Autodesk Fusion 360 part; units mm, degrees
(part 5 of 6)
sketch "taco_truck" plane through (0, 0, 0) normal (0, 1, 0) x (1, 0, 0)
  line L0 (88.25, -7) -> (102.25, -7)
  line L1 (7, -7) -> (7, 7)
  line L2 (83.2, -7) -> (83.2, 7)
  line L3 (-7, 7) -> (-7, -7)
  line L4 (178.45, 7) -> (164.45, 7)
  line L5 (12.05, -7) -> (26.05, -7)
  line L6 (102.25, -7) -> (102.25, 7)
  line L7 (102.25, 7) -> (88.25, 7)
  line L8 (88.25, 7) -> (88.25, -7)
  line L9 (126.35, 7) -> (126.35, -7)
  line L10 (197.5, -7) -> (197.5, 7)
  line L11 (31.1, -7) -> (45.1, -7)
  line L12 (45.1, 7) -> (31.1, 7)
  line L13 (7, 7) -> (-7, 7)
  line L14 (164.45, -7) -> (178.45, -7)
  line L15 (126.35, -7) -> (140.35, -7)
  line L16 (50.15, 7) -> (50.15, -7)
  line L17 (64.15, -7) -> (64.15, 7)
  line L18 (121.3, 7) -> (107.3, 7)
  line L19 (45.1, -7) -> (45.1, 7)
  line L20 (121.3, -7) -> (121.3, 7)
  line L21 (107.3, -7) -> (121.3, -7)
  line L22 (178.45, -7) -> (178.45, 7)
  line L23 (145.4, 7) -> (145.4, -7)
  line L24 (69.2, -7) -> (83.2, -7)
  line L25 (26.05, 7) -> (12.05, 7)
  line L26 (145.4, -7) -> (159.4, -7)
  line L27 (64.15, 7) -> (50.15, 7)
  line L28 (12.05, 7) -> (12.05, -7)
  line L29 (164.45, 7) -> (164.45, -7)
  line L30 (140.35, -7) -> (140.35, 7)
  line L31 (159.4, -7) -> (159.4, 7)
  line L32 (183.5, -7) -> (197.5, -7)
  line L33 (197.5, 7) -> (183.5, 7)
  line L34 (69.2, 7) -> (69.2, -7)
  line L35 (140.35, 7) -> (126.35, 7)
  line L36 (107.3, 7) -> (107.3, -7)
  line L37 (-7, -7) -> (7, -7)
  line L38 (26.05, -7) -> (26.05, 7)
  line L39 (159.4, 7) -> (145.4, 7)
  line L40 (83.2, 7) -> (69.2, 7)
  line L41 (31.1, 7) -> (31.1, -7)
  line L42 (50.15, -7) -> (64.15, -7)
  line L43 (209.6937, -7) -> (223.6938, -7)
  line L44 (183.5, 7) -> (183.5, -7)
  line L45 (209.6937, 7) -> (209.6937, -7)
  line L46 (9.3813, -12.05) -> (-4.6187, -12.05)
  line L47 (-4.6187, -26.05) -> (9.3813, -26.05)
  line L48 (9.3813, -26.05) -> (9.3813, -12.05)
  line L49 (-4.6187, -12.05) -> (-4.6187, -26.05)
  line L50 (16.8125, -26.05) -> (30.8125, -26.05)
  line L51 (30.8125, -12.05) -> (16.8125, -12.05)
  line L52 (223.6938, 7) -> (209.6937, 7)
  line L53 (30.8125, -26.05) -> (30.8125, -12.05)
  line L54 (223.6938, -7) -> (223.6938, 7)
  line L55 (228.4562, -44.013) -> (228.4562, -37.013)
  line L56 (145.1125, -26.05) -> (145.1125, -12.05)
  line L57 (228.4562, -35.575) -> (228.4562, -31.1)
  line L58 (49.8625, -26.05) -> (49.8625, -12.05)
  line L59 (35.8625, -12.05) -> (35.8625, -26.05)
  line L60 (49.8625, -12.05) -> (35.8625, -12.05)
  line L61 (35.8625, -26.05) -> (49.8625, -26.05)
  line L62 (54.9125, -26.05) -> (68.9125, -26.05)
  line L63 (54.9125, -12.05) -> (54.9125, -26.05)
  line L64 (73.9625, -26.05) -> (87.9625, -26.05)
  line L65 (202.2625, -12.05) -> (188.2625, -12.05)
  line L66 (202.2625, -26.05) -> (202.2625, -12.05)
  line L67 (112.0625, -26.05) -> (126.0625, -26.05)
  line L68 (228.4562, -21.575) -> (226.075, -21.575)
  line L69 (214.4563, -26.05) -> (214.4563, -31.1)
  line L70 (59.675, -31.1) -> (59.675, -45.1)
  line L71 (212.075, -12.05) -> (212.075, -26.05)
  line L72 (92.725, -31.1) -> (78.725, -31.1)
  line L73 (21.575, -45.1) -> (35.575, -45.1)
  line L74 (116.825, -45.1) -> (130.825, -45.1)
  line L75 (226.075, -21.575) -> (226.075, -20.137)
  line L76 (150.1625, -26.05) -> (164.1625, -26.05)
  line L77 (78.725, -31.1) -> (78.725, -45.1)
  line L78 (228.4562, -20.137) -> (228.4562, -13.137)
  line L79 (126.0625, -12.05) -> (112.0625, -12.05)
  line L80 (164.1625, -26.05) -> (164.1625, -12.05)
  line L81 (135.875, -45.1) -> (149.875, -45.1)
  line L82 (16.8125, -12.05) -> (16.8125, -26.05)
  line L83 (183.2125, -26.05) -> (183.2125, -12.05)
  line L84 (73.675, -31.1) -> (59.675, -31.1)
  line L85 (169.2125, -12.05) -> (169.2125, -26.05)
  line L86 (228.4562, -13.137) -> (226.075, -13.137)
  line L87 (131.1125, -26.05) -> (145.1125, -26.05)
  line L88 (164.1625, -12.05) -> (150.1625, -12.05)
  line L89 (226.075, -12.05) -> (212.075, -12.05)
  line L90 (87.9625, -12.05) -> (73.9625, -12.05)
  line L91 (107.0125, -12.05) -> (93.0125, -12.05)
  line L92 (228.4562, -31.1) -> (228.4562, -21.575)
  line L93 (93.0125, -26.05) -> (107.0125, -26.05)
  line L94 (212.075, -26.05) -> (214.4562, -26.05)
  line L95 (73.9625, -12.05) -> (73.9625, -26.05)
  line L96 (226.075, -20.137) -> (228.4562, -20.137)
  line L97 (126.0625, -26.05) -> (126.0625, -12.05)
  line L98 (87.9625, -26.05) -> (87.9625, -12.05)
  line L99 (107.0125, -26.05) -> (107.0125, -12.05)
  line L100 (150.1625, -12.05) -> (150.1625, -26.05)
  line L101 (131.1125, -12.05) -> (131.1125, -26.05)
  line L102 (188.2625, -26.05) -> (202.2625, -26.05)
  line L103 (112.0625, -12.05) -> (112.0625, -26.05)
  line L104 (214.4563, -31.1) -> (214.4563, -35.575)
  line L105 (93.0125, -12.05) -> (93.0125, -26.05)
  line L106 (145.1125, -12.05) -> (131.1125, -12.05)
  line L107 (226.075, -13.137) -> (226.075, -12.05)
  line L108 (68.9125, -12.05) -> (54.9125, -12.05)
  line L109 (73.675, -45.1) -> (73.675, -31.1)
  line L110 (183.2125, -12.05) -> (169.2125, -12.05)
  line L111 (97.775, -45.1) -> (111.775, -45.1)
  line L112 (68.9125, -26.05) -> (68.9125, -12.05)
  line L113 (188.2625, -12.05) -> (188.2625, -26.05)
  line L114 (169.2125, -26.05) -> (183.2125, -26.05)
  line L115 (149.875, -45.1) -> (149.875, -31.1)
  line L116 (154.925, -45.1) -> (168.925, -45.1)
  line L117 (187.975, -45.1) -> (187.975, -31.1)
  line L118 (54.625, -31.1) -> (40.625, -31.1)
  line L119 (78.725, -45.1) -> (92.725, -45.1)
  line L120 (11.7625, -45.1) -> (11.7625, -31.1)
  line L121 (47.7688, -64.15) -> (48.8875, -64.15)
  line L122 (97.775, -31.1) -> (97.775, -45.1)
  line L123 (214.4563, -37.013) -> (213.4563, -37.013)
  line L124 (-2.2375, -31.1) -> (-2.2375, -45.1)
  line L125 (134.6442, -64.15) -> (141.6442, -64.15)
  line L126 (173.975, -45.1) -> (187.975, -45.1)
  line L127 (228.4562, -37.013) -> (228.4562, -35.575)
  line L128 (207.025, -31.1) -> (193.025, -31.1)
  line L129 (213.4562, -44.013) -> (214.4563, -44.013)
  line L130 (213.4562, -37.013) -> (213.4562, -44.013)
  line L131 (173.975, -31.1) -> (173.975, -45.1)
  line L132 (154.925, -31.1) -> (154.925, -45.1)
  line L133 (-2.2375, -45.1) -> (11.7625, -45.1)
  line L134 (168.925, -31.1) -> (154.925, -31.1)
  line L135 (-4.6187, -64.15) -> (9.3813, -64.15)
  line L136 (35.575, -31.1) -> (21.575, -31.1)
  line L137 (193.025, -45.1) -> (207.025, -45.1)
  line L138 (92.725, -45.1) -> (92.725, -31.1)
  line L139 (21.575, -31.1) -> (21.575, -45.1)
  line L140 (35.575, -45.1) -> (35.575, -31.1)
  line L141 (11.7625, -31.1) -> (-2.2375, -31.1)
  line L142 (197.7875, -64.15) -> (211.7875, -64.15)
  line L143 (214.4563, -35.575) -> (214.4563, -37.013)
  line L144 (168.925, -45.1) -> (168.925, -31.1)
  line L145 (178.7375, -50.15) -> (178.7375, -64.15)
  line L146 (21.575, -50.15) -> (21.575, -64.15)
  line L147 (197.7875, -50.15) -> (197.7875, -64.15)
  line L148 (35.575, -64.15) -> (35.575, -50.15)
  line L149 (61.7688, -64.15) -> (61.7688, -50.15)
  line L150 (207.025, -45.1) -> (207.025, -31.1)
  line L151 (9.3813, -50.15) -> (-4.6187, -50.15)
  line L152 (54.625, -45.1) -> (54.625, -31.1)
  line L153 (40.625, -31.1) -> (40.625, -45.1)
  line L154 (111.775, -31.1) -> (97.775, -31.1)
  line L155 (135.875, -31.1) -> (135.875, -45.1)
  line L156 (187.975, -31.1) -> (173.975, -31.1)
  line L157 (130.825, -31.1) -> (116.825, -31.1)
  line L158 (193.025, -31.1) -> (193.025, -45.1)
  line L159 (9.3813, -64.15) -> (9.3813, -50.15)
  line L160 (214.4563, -44.013) -> (214.4563, -45.1)
  line L161 (228.4562, -45.1) -> (228.4562, -44.013)
  line L162 (111.775, -45.1) -> (111.775, -31.1)
  line L163 (214.4563, -45.1) -> (228.4563, -45.1)
  line L164 (130.825, -45.1) -> (130.825, -31.1)
  line L165 (116.825, -31.1) -> (116.825, -45.1)
  line L166 (21.575, -64.15) -> (35.575, -64.15)
  line L167 (59.675, -45.1) -> (73.675, -45.1)
  line L168 (-4.6187, -50.15) -> (-4.6187, -64.15)
  line L169 (35.575, -50.15) -> (21.575, -50.15)
  line L170 (48.8875, -64.15) -> (55.8875, -64.15)
  line L171 (55.8875, -64.15) -> (61.7688, -64.15)
  line L172 (40.625, -45.1) -> (54.625, -45.1)
  line L173 (149.875, -31.1) -> (135.875, -31.1)
  line L174 (230.8375, -50.15) -> (216.8375, -50.15)
  line L175 (61.7688, -50.15) -> (55.8875, -50.15)
  line L176 (55.8875, -50.15) -> (55.8875, -49.15)
  line L177 (117.7683, -49.15) -> (110.7682, -49.15)
  line L178 (163.1875, -50.15) -> (154.925, -50.15)
  line L179 (134.6442, -49.15) -> (134.6442, -64.15)
  line L180 (116.5375, -64.15) -> (117.7683, -64.15)
  line L181 (102.5375, -64.15) -> (110.7682, -64.15)
  line L182 (163.1875, -64.15) -> (168.925, -64.15)
  line L183 (192.7375, -64.15) -> (192.7375, -50.15)
  line L184 (110.7682, -49.15) -> (110.7682, -50.15)
  line L185 (178.7375, -64.15) -> (192.7375, -64.15)
  line L186 (111.775, -64.15) -> (116.5375, -64.15)
  line L187 (230.8375, -64.15) -> (230.8375, -50.15)
  line L188 (102.5375, -50.15) -> (101.163, -50.15)
  line L189 (101.163, -50.15) -> (101.163, -49.15)
  line L190 (110.7682, -50.15) -> (102.5375, -50.15)
  line L191 (119.2062, -64.15) -> (133.2063, -64.15)
  line L192 (117.7683, -64.15) -> (117.7683, -49.15)
  line L193 (77.287, -64.15) -> (77.287, -49.15)
  line L194 (154.925, -50.15) -> (154.925, -64.15)
  line L195 (141.6442, -49.15) -> (134.6442, -49.15)
  line L196 (211.7875, -64.15) -> (211.7875, -50.15)
  line L197 (48.8875, -50.15) -> (47.7688, -50.15)
  line L198 (119.2062, -50.15) -> (119.2062, -64.15)
  line L199 (216.8375, -50.15) -> (216.8375, -64.15)
  line L200 (133.2063, -64.15) -> (133.2063, -50.15)
  line L201 (97.775, -64.15) -> (101.163, -64.15)
  line L202 (78.725, -50.15) -> (78.725, -64.15)
  line L203 (78.725, -64.15) -> (92.725, -64.15)
  line L204 (47.7688, -50.15) -> (47.7688, -64.15)
  line L205 (92.725, -50.15) -> (78.725, -50.15)
  line L206 (101.163, -49.15) -> (94.163, -49.15)
  line L207 (170.1875, -49.15) -> (163.1875, -49.15)
  line L208 (163.1875, -49.15) -> (163.1875, -50.15)
  line L209 (70.287, -64.15) -> (77.287, -64.15)
  line L210 (170.1875, -64.15) -> (170.1875, -49.15)
  line L211 (92.725, -64.15) -> (92.725, -50.15)
  line L212 (77.287, -49.15) -> (70.287, -49.15)
  line L213 (110.7682, -64.15) -> (111.775, -64.15)
  line L214 (211.7875, -50.15) -> (197.7875, -50.15)
  line L215 (192.7375, -50.15) -> (178.7375, -50.15)
  line L216 (48.8875, -49.15) -> (48.8875, -50.15)
  line L217 (55.8875, -49.15) -> (48.8875, -49.15)
  line L218 (70.287, -49.15) -> (70.287, -64.15)
  line L219 (216.8375, -64.15) -> (230.8375, -64.15)
  line L220 (141.6442, -64.15) -> (141.6442, -49.15)
  line L221 (101.163, -64.15) -> (102.5375, -64.15)
  line L222 (94.163, -49.15) -> (94.163, -64.15)
  line L223 (94.163, -64.15) -> (97.775, -64.15)
  line L224 (154.925, -64.15) -> (163.1875, -64.15)
  line L225 (168.925, -64.15) -> (170.1875, -64.15)
  line L226 (133.2063, -50.15) -> (119.2063, -50.15)
sketch "wanten" plane through (0, 0, 0) normal (0, 1, 0) x (1, 0, 0)
  line L0 (50.15, -45.1) -> (64.15, -45.1)
  line L1 (64.15, -45.1) -> (64.15, -31.1)
  line L2 (45.1, -45.1) -> (45.1, -31.1)
  line L3 (45.1, -31.1) -> (31.1, -31.1)
  line L4 (69.2, -26.05) -> (83.2, -26.05)
  line L5 (197.7875, -12.05) -> (197.7875, -26.05)
  line L6 (159.6875, -12.05) -> (159.6875, -26.05)
  line L7 (178.7375, -12.05) -> (178.7375, -26.05)
  line L8 (64.15, -31.1) -> (50.15, -31.1)
  line L9 (31.1, -31.1) -> (31.1, -45.1)
  line L10 (197.7875, -26.05) -> (211.7875, -26.05)
  line L11 (192.7375, -26.05) -> (192.7375, -12.05)
  line L12 (12.05, -45.1) -> (26.05, -45.1)
  line L13 (140.6375, -12.05) -> (140.6375, -26.05)
  line L14 (7, -45.1) -> (7, -31.1)
  line L15 (-7, -45.1) -> (7, -45.1)
  line L16 (7, -31.1) -> (-7, -31.1)
  line L17 (211.7875, -12.05) -> (197.7875, -12.05)
  line L18 (211.7875, -26.05) -> (211.7875, -12.05)
  line L19 (-7, -31.1) -> (-7, -45.1)
  line L20 (26.05, -45.1) -> (26.05, -31.1)
  line L21 (12.05, -31.1) -> (12.05, -45.1)
  line L22 (31.1, -45.1) -> (45.1, -45.1)
  line L23 (114.4438, -12.05) -> (114.4438, -26.05)
  line L24 (26.05, -31.1) -> (12.05, -31.1)
  line L25 (178.7375, -26.05) -> (192.7375, -26.05)
  line L26 (192.7375, -12.05) -> (178.7375, -12.05)
  line L27 (45.1, 7) -> (31.1, 7)
  line L28 (173.6875, -12.05) -> (159.6875, -12.05)
  line L29 (83.2, -26.05) -> (83.2, -12.05)
  line L30 (230.8375, -26.05) -> (230.8375, -12.05)
  line L31 (230.8375, -12.05) -> (216.8375, -12.05)
  line L32 (154.6375, -26.05) -> (154.6375, -12.05)
  line L33 (83.2, -12.05) -> (69.2, -12.05)
  line L34 (128.4437, -12.05) -> (114.4438, -12.05)
  line L35 (102.25, -26.05) -> (102.25, -12.05)
  line L36 (88.25, -12.05) -> (88.25, -26.05)
  line L37 (154.6375, -12.05) -> (140.6375, -12.05)
  line L38 (7, 7) -> (-7, 7)
  line L39 (12.05, -7) -> (26.05, -7)
  line L40 (211.7875, 7) -> (197.7875, 7)
  line L41 (26.05, -7) -> (26.05, 7)
  line L42 (45.1, -7) -> (45.1, 7)
  line L43 (216.8375, -12.05) -> (216.8375, -26.05)
  line L44 (-7, -7) -> (7, -7)
  line L45 (88.25, -7) -> (102.25, -7)
  line L46 (128.4437, -7) -> (128.4437, 7)
  line L47 (154.6375, -7) -> (154.6375, 7)
  line L48 (7, -7) -> (7, 7)
  line L49 (102.25, 7) -> (88.25, 7)
  line L50 (102.25, -12.05) -> (88.25, -12.05)
  line L51 (114.4438, -26.05) -> (128.4437, -26.05)
  line L52 (-7, 7) -> (-7, -7)
  line L53 (102.25, -7) -> (102.25, 7)
  line L54 (64.15, 7) -> (50.15, 7)
  line L55 (140.6375, -26.05) -> (154.6375, -26.05)
  line L56 (197.7875, -7) -> (211.7875, -7)
  line L57 (12.05, 7) -> (12.05, -7)
  line L58 (159.6875, -26.05) -> (173.6875, -26.05)
  line L59 (114.4438, -7) -> (128.4437, -7)
  line L60 (31.1, 7) -> (31.1, -7)
  line L61 (216.8375, -26.05) -> (230.8375, -26.05)
  line L62 (69.2, 7) -> (69.2, -7)
  line L63 (64.15, -7) -> (64.15, 7)
  line L64 (69.2, -12.05) -> (69.2, -26.05)
  line L65 (154.6375, 7) -> (140.6375, 7)
  line L66 (128.4437, 7) -> (114.4438, 7)
  line L67 (140.6375, 7) -> (140.6375, -7)
  line L68 (83.2, -7) -> (83.2, 7)
  line L69 (173.6875, 7) -> (159.6875, 7)
  line L70 (173.6875, -7) -> (173.6875, 7)
  line L71 (128.4437, -26.05) -> (128.4437, -12.05)
  line L72 (83.2, 7) -> (69.2, 7)
  line L73 (69.2, -7) -> (83.2, -7)
  line L74 (159.6875, -7) -> (173.6875, -7)
  line L75 (31.1, -7) -> (45.1, -7)
  line L76 (173.6875, -26.05) -> (173.6875, -12.05)
  line L77 (88.25, -26.05) -> (102.25, -26.05)
  line L78 (140.6375, -7) -> (154.6375, -7)
  line L79 (26.05, 7) -> (12.05, 7)
  line L80 (50.15, -12.05) -> (50.15, -26.05)
  line L81 (93.0125, -50.15) -> (91.5745, -50.15)
  line L82 (102.25, -31.1) -> (88.25, -31.1)
  line L83 (159.6875, -31.1) -> (159.6875, -45.1)
  line L84 (216.8375, -45.1) -> (230.8375, -45.1)
  line L85 (159.6875, 7) -> (159.6875, -7)
  line L86 (31.1, -12.05) -> (31.1, -26.05)
  line L87 (12.05, -12.05) -> (12.05, -26.05)
  line L88 (216.8375, -7) -> (230.8375, -7)
  line L89 (91.5745, -64.15) -> (93.0125, -64.15)
  line L90 (211.7875, -31.1) -> (197.7875, -31.1)
  line L91 (128.4437, -45.1) -> (128.4437, -31.1)
  line L92 (114.4438, 7) -> (114.4438, -7)
  line L93 (-4.6187, -64.15) -> (9.3813, -64.15)
  line L94 (197.7875, 7) -> (197.7875, -7)
  line L95 (114.4438, -31.1) -> (114.4438, -45.1)
  line L96 (178.7375, 7) -> (178.7375, -7)
  line L97 (178.7375, -7) -> (192.7375, -7)
  line L98 (7, -12.05) -> (-7, -12.05)
  line L99 (26.05, -26.05) -> (26.05, -12.05)
  line L100 (140.6375, -31.1) -> (140.6375, -45.1)
  line L101 (192.7375, -45.1) -> (192.7375, -31.1)
  line L102 (108.4505, -49.15) -> (106.0375, -49.15)
  line L103 (64.15, -12.05) -> (50.15, -12.05)
  line L104 (107.0125, -64.15) -> (108.4505, -64.15)
  line L105 (112.0625, -64.15) -> (113.0375, -64.15)
  line L106 (33.1938, -50.15) -> (19.1938, -50.15)
  line L107 (88.25, 7) -> (88.25, -7)
  line L108 (93.0125, -64.15) -> (97.4875, -64.15)
  line L109 (-7, -12.05) -> (-7, -26.05)
  line L110 (64.15, -26.05) -> (64.15, -12.05)
  line L111 (31.1, -26.05) -> (45.1, -26.05)
  line L112 (45.1, -12.05) -> (31.1, -12.05)
  line L113 (50.15, -7) -> (64.15, -7)
  line L114 (216.8375, 7) -> (216.8375, -7)
  line L115 (33.1938, -64.15) -> (33.1938, -50.15)
  line L116 (83.2, -45.1) -> (83.2, -31.1)
  line L117 (69.2, -45.1) -> (83.2, -45.1)
  line L118 (-7, -26.05) -> (7, -26.05)
  line L119 (230.8375, -7) -> (230.8375, 7)
  line L120 (102.25, -45.1) -> (102.25, -31.1)
  line L121 (106.0375, -49.15) -> (106.0375, -50.15)
  line L122 (26.05, -12.05) -> (12.05, -12.05)
  line L123 (192.7375, 7) -> (178.7375, 7)
  line L124 (192.7375, -7) -> (192.7375, 7)
  line L125 (230.8375, 7) -> (216.8375, 7)
  line L126 (12.05, -26.05) -> (26.05, -26.05)
  line L127 (50.15, -26.05) -> (64.15, -26.05)
  line L128 (50.15, 7) -> (50.15, -7)
  line L129 (192.7375, -31.1) -> (178.7375, -31.1)
  line L130 (178.7375, -45.1) -> (192.7375, -45.1)
  line L131 (88.25, -31.1) -> (88.25, -45.1)
  line L132 (45.1, -26.05) -> (45.1, -12.05)
  line L133 (114.4438, -45.1) -> (128.4437, -45.1)
  line L134 (211.7875, -7) -> (211.7875, 7)
  line L135 (74.9375, -49.15) -> (67.9438, -49.15)
  line L136 (154.6375, -31.1) -> (140.6375, -31.1)
  line L137 (140.6375, -45.1) -> (154.6375, -45.1)
  line L138 (197.7875, -45.1) -> (211.7875, -45.1)
  line L139 (154.6375, -45.1) -> (154.6375, -31.1)
  line L140 (216.8375, -31.1) -> (216.8375, -45.1)
  line L141 (7, -26.05) -> (7, -12.05)
  line L142 (84.4625, -50.15) -> (84.4625, -49.15)
  line L143 (163.1875, -49.15) -> (163.1875, -64.15)
  line L144 (67.9375, -49.15) -> (67.9375, -50.15)
  line L145 (159.6875, -45.1) -> (173.6875, -45.1)
  line L146 (230.8375, -31.1) -> (216.8375, -31.1)
  line L147 (83.2, -31.1) -> (69.2, -31.1)
  line L148 (140.6375, -50.15) -> (133.4938, -50.15)
  line L149 (155.9317, -49.15) -> (148.9317, -49.15)
  line L150 (154.6375, -64.15) -> (155.9317, -64.15)
  line L151 (115.4505, -49.15) -> (113.0375, -49.15)
  line L152 (115.4505, -64.15) -> (125.0558, -64.15)
  line L153 (57.0063, -50.15) -> (43.0063, -50.15)
  line L154 (197.7875, -31.1) -> (197.7875, -45.1)
  line L155 (69.2, -31.1) -> (69.2, -45.1)
  line L156 (91.5745, -50.15) -> (91.5745, -49.15)
  line L157 (179.7125, -49.15) -> (174.9438, -49.15)
  line L158 (147.4938, -50.15) -> (140.6375, -50.15)
  line L159 (125.0875, -64.15) -> (126.0625, -64.15)
  line L160 (50.15, -31.1) -> (50.15, -45.1)
  line L161 (163.1875, -64.15) -> (164.45, -64.15)
  line L162 (43.0063, -64.15) -> (57.0063, -64.15)
  line L163 (125.0875, -49.15) -> (125.0557, -49.15)
  line L164 (83.4875, -64.15) -> (84.4625, -64.15)
  line L165 (84.4625, -49.15) -> (77.4625, -49.15)
  line L166 (230.8375, -45.1) -> (230.8375, -31.1)
  line L167 (211.7875, -45.1) -> (211.7875, -31.1)
  line L168 (84.5745, -64.15) -> (91.5745, -64.15)
  line L169 (128.4437, -31.1) -> (114.4438, -31.1)
  line L170 (173.6875, -31.1) -> (159.6875, -31.1)
  line L171 (178.7375, -64.15) -> (179.7125, -64.15)
  line L172 (179.7125, -50.15) -> (179.7125, -49.15)
  line L173 (97.4875, -50.15) -> (93.0125, -50.15)
  line L174 (77.4625, -49.15) -> (77.4625, -50.15)
  line L175 (167.9437, -49.15) -> (163.1875, -49.15)
  line L176 (132.0875, -49.15) -> (132.0558, -49.15)
  line L177 (108.4505, -64.15) -> (112.0625, -64.15)
  line L178 (9.3813, -64.15) -> (9.3813, -50.15)
  line L179 (148.9317, -50.15) -> (147.4938, -50.15)
  line L180 (84.4625, -64.15) -> (84.5745, -64.15)
  line L181 (132.0557, -49.15) -> (125.0875, -49.15)
  line L182 (133.4938, -64.15) -> (140.6375, -64.15)
  line L183 (178.7375, -31.1) -> (178.7375, -45.1)
  line L184 (-4.6187, -50.15) -> (-4.6187, -64.15)
  line L185 (174.9438, -64.15) -> (178.45, -64.15)
  line L186 (77.4625, -50.15) -> (74.9438, -50.15)
  line L187 (9.3813, -50.15) -> (-4.6187, -50.15)
  line L188 (74.9375, -64.15) -> (74.9438, -64.15)
  line L189 (19.1938, -64.15) -> (33.1938, -64.15)
  line L190 (113.0375, -64.15) -> (114.4438, -64.15)
  line L191 (64.4375, -64.15) -> (67.9375, -64.15)
  line L192 (43.0063, -50.15) -> (43.0063, -64.15)
  line L193 (67.9375, -64.15) -> (67.9438, -64.15)
  line L194 (155.9317, -64.15) -> (155.9317, -49.15)
  line L195 (173.6875, -45.1) -> (173.6875, -31.1)
  line L196 (67.9438, -64.15) -> (74.9375, -64.15)
  line L197 (88.25, -45.1) -> (102.25, -45.1)
  line L198 (67.9438, -49.15) -> (67.9375, -49.15)
  line L199 (84.5745, -50.15) -> (84.4625, -50.15)
  line L200 (113.0375, -49.15) -> (108.4505, -49.15)
  line L201 (19.1938, -50.15) -> (19.1938, -64.15)
  line L202 (106.0375, -64.15) -> (107.0125, -64.15)
  line L203 (57.0063, -64.15) -> (57.0063, -50.15)
  line L204 (114.4438, -64.15) -> (115.4505, -64.15)
  line L205 (91.5745, -49.15) -> (84.5745, -49.15)
  line L206 (132.0557, -64.15) -> (132.0875, -64.15)
  line L207 (170.1875, -64.15) -> (172.7125, -64.15)
  line L208 (125.0557, -49.15) -> (125.0557, -50.15)
  line L209 (78.4375, -64.15) -> (83.4875, -64.15)
  line L210 (197.7875, -64.15) -> (199.8812, -64.15)
  line L211 (216.8375, -50.15) -> (212.075, -50.15)
  line L212 (185.8813, -64.15) -> (192.7375, -64.15)
  line L213 (174.9438, -49.15) -> (172.7125, -49.15)
  line L214 (148.9317, -64.15) -> (154.6375, -64.15)
  line L215 (212.075, -64.15) -> (216.8375, -64.15)
  line L216 (148.9317, -49.15) -> (148.9317, -50.15)
  line L217 (226.075, -50.15) -> (221.3125, -50.15)
  line L218 (199.8812, -50.15) -> (197.7875, -50.15)
  line L219 (115.4505, -50.15) -> (115.4505, -49.15)
  line L220 (125.0557, -64.15) -> (125.0875, -64.15)
  line L221 (170.1875, -49.15) -> (167.9437, -49.15)
  line L222 (167.9437, -64.15) -> (170.1875, -64.15)
  line L223 (192.7375, -64.15) -> (197.7875, -64.15)
  line L224 (207.3125, -50.15) -> (199.8812, -50.15)
  line L225 (128.4437, -64.15) -> (132.0557, -64.15)
  line L226 (132.0875, -64.15) -> (132.0875, -49.15)
  line L227 (74.9438, -49.15) -> (74.9375, -49.15)
  line L228 (77.4625, -64.15) -> (78.4375, -64.15)
  line L229 (133.4938, -50.15) -> (133.4938, -64.15)
  line L230 (84.5745, -49.15) -> (84.5745, -50.15)
  line L231 (64.4375, -50.15) -> (64.4375, -64.15)
  line L232 (226.075, -64.15) -> (230.8375, -64.15)
  line L233 (211.7875, -64.15) -> (212.075, -64.15)
  line L234 (207.3125, -64.15) -> (211.7875, -64.15)
  line L235 (211.7875, -50.15) -> (207.3125, -50.15)
  line L236 (192.7375, -50.15) -> (185.8813, -50.15)
  line L237 (106.0375, -50.15) -> (97.4875, -50.15)
  line L238 (172.7125, -64.15) -> (174.9438, -64.15)
  line L239 (172.7125, -49.15) -> (170.1875, -49.15)
  line L240 (147.4938, -64.15) -> (148.9317, -64.15)
  line L241 (179.7125, -64.15) -> (185.8813, -64.15)
  line L242 (212.075, -50.15) -> (211.7875, -50.15)
  line L243 (197.7875, -50.15) -> (192.7375, -50.15)
  line L244 (178.45, -64.15) -> (178.7375, -64.15)
  line L245 (126.0625, -64.15) -> (128.4437, -64.15)
  line L246 (125.0557, -50.15) -> (115.4505, -50.15)
  line L247 (74.9438, -64.15) -> (77.4625, -64.15)
  line L248 (140.6375, -64.15) -> (147.4938, -64.15)
  line L249 (67.9375, -50.15) -> (64.4375, -50.15)
  line L250 (221.3125, -50.15) -> (216.8375, -50.15)
  line L251 (97.4875, -64.15) -> (106.0375, -64.15)
  line L252 (74.9438, -50.15) -> (74.9438, -49.15)
  line L253 (230.8375, -64.15) -> (230.8375, -50.15)
  line L254 (216.8375, -64.15) -> (221.3125, -64.15)
  line L255 (164.45, -64.15) -> (167.9437, -64.15)
  line L256 (185.8813, -50.15) -> (179.7125, -50.15)
  line L257 (230.8375, -50.15) -> (226.075, -50.15)
  line L258 (221.3125, -64.15) -> (226.075, -64.15)
  line L259 (199.8812, -64.15) -> (207.3125, -64.15)
  line L260 (-7, 7) -> (7, -7) construction
  constraint midpoint L260 origin
extrude "Extrude9" cut sketch "wanten" along normal blind 10 bodies 1 2 3 4 5
sketch "plate_campiander" plane through (0, 10, 0) normal (0, 1, 0) x (-1, 0, 0)
  line L0 (-220.1576, 71.15) -> (-222.6139, 71.15)
  arc A0 (-223.1114, 71.15) -> (-222.6139, 71.15) centre (-222.8626, 69.925) ccw
  line L1 (-223.1114, 71.15) -> (-228.2294, 71.15)
  line L2 (-228.2294, 71.15) -> (-230.5388, 67.15)
  arc A1 (-232.2709, 66.15) -> (-230.5388, 67.15) centre (-232.2709, 68.15) ccw
  line L3 (-232.2709, 66.15) -> (-232.3375, 66.15)
  arc A2 (-232.3375, 66.15) -> (-232.8375, 65.65) centre (-232.3375, 65.65) ccw
  line L4 (-232.8375, 65.65) -> (-232.8375, -8.5)
  arc A3 (-232.8375, -8.5) -> (-232.3375, -9) centre (-232.3375, -8.5) ccw
  line L5 (-232.3375, -9) -> (-232.2709, -9)
  arc A4 (-230.5388, -10) -> (-232.2709, -9) centre (-232.2709, -11) ccw
  line L6 (-230.5388, -10) -> (-228.2294, -14)
  line L7 (-228.2294, -14) -> (-223.1111, -14)
  arc A5 (-222.6136, -14) -> (-223.1111, -14) centre (-222.8624, -12.775) ccw
  line L8 (-222.6136, -14) -> (-220.1576, -14)
  line L9 (-220.1576, -14) -> (-217.8482, -10)
  arc A6 (-216.1161, -9) -> (-217.8482, -10) centre (-216.1161, -11) ccw
  line L10 (-216.1161, -9) -> (-7.7214, -9)
  arc A7 (-5.9893, -10) -> (-7.7214, -9) centre (-7.7214, -11) ccw
  line L11 (-5.9893, -10) -> (-3.6799, -14)
  line L12 (-3.6799, -14) -> (-1.2236, -14)
  arc A8 (-0.7261, -14) -> (-1.2236, -14) centre (-0.9749, -12.775) ccw
  line L13 (-0.7261, -14) -> (4.3919, -14)
  line L14 (4.3919, -14) -> (6.7013, -10)
  arc A9 (8.4334, -9) -> (6.7013, -10) centre (8.4334, -11) ccw
  line L15 (8.4334, -9) -> (8.5, -9)
  arc A10 (8.5, -9) -> (9, -8.5) centre (8.5, -8.5) ccw
  line L16 (9, -8.5) -> (9, 65.65)
  arc A11 (9, 65.65) -> (8.5, 66.15) centre (8.5, 65.65) ccw
  line L17 (8.5, 66.15) -> (8.4334, 66.15)
  arc A12 (6.7013, 67.15) -> (8.4334, 66.15) centre (8.4334, 68.15) ccw
  line L18 (6.7013, 67.15) -> (4.3919, 71.15)
  line L19 (4.3919, 71.15) -> (-0.7264, 71.15)
  arc A13 (-1.2239, 71.15) -> (-0.7264, 71.15) centre (-0.9751, 69.925) ccw
  line L20 (-1.2239, 71.15) -> (-3.6799, 71.15)
  line L21 (-3.6799, 71.15) -> (-5.9893, 67.15)
  arc A14 (-7.7214, 66.15) -> (-5.9893, 67.15) centre (-7.7214, 68.15) ccw
  line L22 (-7.7214, 66.15) -> (-216.1161, 66.15)
  arc A15 (-217.8482, 67.15) -> (-216.1161, 66.15) centre (-216.1161, 68.15) ccw
  line L23 (-217.8482, 67.15) -> (-220.1576, 71.15)
  line L24 (-88.25, 26.05) -> (-88.25, 12.05)
  line L25 (-88.25, 12.05) -> (-102.25, 12.05)
  line L26 (-102.25, 12.05) -> (-102.25, 26.05)
  line L27 (-102.25, 26.05) -> (-88.25, 26.05)
  line L28 (-230.8375, 45.1) -> (-216.8375, 45.1)
  line L29 (-216.8375, 45.1) -> (-216.8375, 31.1)
  line L30 (-216.8375, 31.1) -> (-230.8375, 31.1)
  line L31 (-230.8375, 31.1) -> (-230.8375, 45.1)
  line L32 (-50.15, 31.1) -> (-64.15, 31.1)
  line L33 (-64.15, 31.1) -> (-64.15, 45.1)
  line L34 (-64.15, 45.1) -> (-50.15, 45.1)
  line L35 (-50.15, 45.1) -> (-50.15, 31.1)
  line L36 (-57.0063, 64.15) -> (-43.0063, 64.15)
  line L37 (-43.0063, 64.15) -> (-43.0063, 50.15)
  line L38 (-43.0063, 50.15) -> (-57.0063, 50.15)
  line L39 (-57.0063, 50.15) -> (-57.0063, 64.15)
  line L40 (-140.6375, 26.05) -> (-140.6375, 12.05)
  line L41 (-140.6375, 12.05) -> (-154.6375, 12.05)
  line L42 (-154.6375, 12.05) -> (-154.6375, 26.05)
  line L43 (-154.6375, 26.05) -> (-140.6375, 26.05)
  line L44 (-230.8375, -7) -> (-230.8375, 7)
  line L45 (-230.8375, 7) -> (-216.8375, 7)
  line L46 (-216.8375, 7) -> (-216.8375, -7)
  line L47 (-216.8375, -7) -> (-230.8375, -7)
  line L48 (-31.1, 7) -> (-31.1, -7)
  line L49 (-31.1, -7) -> (-45.1, -7)
  line L50 (-45.1, -7) -> (-45.1, 7)
  line L51 (-45.1, 7) -> (-31.1, 7)
  line L52 (-211.7875, 45.1) -> (-197.7875, 45.1)
  line L53 (-197.7875, 45.1) -> (-197.7875, 31.1)
  line L54 (-197.7875, 31.1) -> (-211.7875, 31.1)
  line L55 (-211.7875, 31.1) -> (-211.7875, 45.1)
  line L56 (-12.05, 26.05) -> (-12.05, 12.05)
  line L57 (-12.05, 12.05) -> (-26.05, 12.05)
  line L58 (-26.05, 12.05) -> (-26.05, 26.05)
  line L59 (-26.05, 26.05) -> (-12.05, 26.05)
  line L60 (-26.05, -7) -> (-26.05, 7)
  line L61 (-26.05, 7) -> (-12.05, 7)
  line L62 (-12.05, 7) -> (-12.05, -7)
  line L63 (-12.05, -7) -> (-26.05, -7)
  line L64 (-128.4437, 31.1) -> (-128.4437, 45.1)
  line L65 (-128.4437, 45.1) -> (-114.4438, 45.1)
  line L66 (-114.4438, 45.1) -> (-114.4438, 31.1)
  line L67 (-114.4438, 31.1) -> (-128.4437, 31.1)
  line L68 (-140.6375, 7) -> (-140.6375, -7)
  line L69 (-140.6375, -7) -> (-154.6375, -7)
  line L70 (-154.6375, -7) -> (-154.6375, 7)
  line L71 (-154.6375, 7) -> (-140.6375, 7)
  line L72 (-192.7375, 12.05) -> (-192.7375, 26.05)
  line L73 (-192.7375, 26.05) -> (-178.7375, 26.05)
  line L74 (-178.7375, 26.05) -> (-178.7375, 12.05)
  line L75 (-178.7375, 12.05) -> (-192.7375, 12.05)
  line L76 (-173.6875, 45.1) -> (-159.6875, 45.1)
  line L77 (-159.6875, 45.1) -> (-159.6875, 31.1)
  line L78 (-159.6875, 31.1) -> (-173.6875, 31.1)
  line L79 (-173.6875, 31.1) -> (-173.6875, 45.1)
  line L80 (-159.6875, -7) -> (-173.6875, -7)
  line L81 (-173.6875, -7) -> (-173.6875, 7)
  line L82 (-173.6875, 7) -> (-159.6875, 7)
  line L83 (-159.6875, 7) -> (-159.6875, -7)
  line L84 (-50.15, 26.05) -> (-50.15, 12.05)
  line L85 (-50.15, 12.05) -> (-64.15, 12.05)
  line L86 (-64.15, 12.05) -> (-64.15, 26.05)
  line L87 (-64.15, 26.05) -> (-50.15, 26.05)
  line L88 (-19.1938, 50.15) -> (-33.1938, 50.15)
  line L89 (-33.1938, 50.15) -> (-33.1938, 64.15)
  line L90 (-33.1938, 64.15) -> (-19.1938, 64.15)
  line L91 (-19.1938, 64.15) -> (-19.1938, 50.15)
  line L92 (-192.7375, 7) -> (-178.7375, 7)
  line L93 (-178.7375, 7) -> (-178.7375, -7)
  line L94 (-178.7375, -7) -> (-192.7375, -7)
  line L95 (-192.7375, -7) -> (-192.7375, 7)
  line L96 (-69.2, 7) -> (-69.2, -7)
  line L97 (-69.2, -7) -> (-83.2, -7)
  line L98 (-83.2, -7) -> (-83.2, 7)
  line L99 (-83.2, 7) -> (-69.2, 7)
  line L100 (-133.4938, 64.15) -> (-133.4938, 50.15)
  line L101 (-133.4938, 50.15) -> (-148.9318, 50.15)
  line L102 (-148.9317, 50.15) -> (-148.9317, 49.15)
  line L103 (-148.9317, 49.15) -> (-155.9317, 49.15)
  line L104 (-155.9317, 49.15) -> (-155.9317, 64.15)
  line L105 (-155.9317, 64.15) -> (-133.4938, 64.15)
  line L106 (-88.25, -7) -> (-102.25, -7)
  line L107 (-102.25, -7) -> (-102.25, 7)
  line L108 (-102.25, 7) -> (-88.25, 7)
  line L109 (-88.25, 7) -> (-88.25, -7)
  line L110 (-211.7875, 7) -> (-197.7875, 7)
  line L111 (-197.7875, 7) -> (-197.7875, -7)
  line L112 (-197.7875, -7) -> (-211.7875, -7)
  line L113 (-211.7875, -7) -> (-211.7875, 7)
  line L114 (-173.6875, 26.05) -> (-159.6875, 26.05)
  line L115 (-159.6875, 26.05) -> (-159.6875, 12.05)
  line L116 (-159.6875, 12.05) -> (-173.6875, 12.05)
  line L117 (-173.6875, 12.05) -> (-173.6875, 26.05)
  line L118 (-50.15, -7) -> (-64.15, -7)
  line L119 (-64.15, -7) -> (-64.15, 7)
  line L120 (-64.15, 7) -> (-50.15, 7)
  line L121 (-50.15, 7) -> (-50.15, -7)
  line L122 (-216.8375, 26.05) -> (-216.8375, 12.05)
  line L123 (-216.8375, 12.05) -> (-230.8375, 12.05)
  line L124 (-230.8375, 12.05) -> (-230.8375, 26.05)
  line L125 (-230.8375, 26.05) -> (-216.8375, 26.05)
  line L126 (-128.4437, 26.05) -> (-114.4438, 26.05)
  line L127 (-114.4438, 26.05) -> (-114.4438, 12.05)
  line L128 (-114.4438, 12.05) -> (-128.4437, 12.05)
  line L129 (-128.4437, 12.05) -> (-128.4437, 26.05)
  line L130 (-154.6375, 45.1) -> (-140.6375, 45.1)
  line L131 (-140.6375, 45.1) -> (-140.6375, 31.1)
  line L132 (-140.6375, 31.1) -> (-154.6375, 31.1)
  line L133 (-154.6375, 31.1) -> (-154.6375, 45.1)
  line L134 (-69.2, 12.05) -> (-83.2, 12.05)
  line L135 (-83.2, 12.05) -> (-83.2, 26.05)
  line L136 (-83.2, 26.05) -> (-69.2, 26.05)
  line L137 (-69.2, 26.05) -> (-69.2, 12.05)
  line L138 (-178.7375, 31.1) -> (-192.7375, 31.1)
  line L139 (-192.7375, 31.1) -> (-192.7375, 45.1)
  line L140 (-192.7375, 45.1) -> (-178.7375, 45.1)
  line L141 (-178.7375, 45.1) -> (-178.7375, 31.1)
  line L142 (7, -7) -> (-7, -7)
  line L143 (-7, -7) -> (-7, 7)
  line L144 (-7, 7) -> (7, 7)
  line L145 (7, 7) -> (7, -7)
  line L146 (-45.1, 26.05) -> (-31.1, 26.05)
  line L147 (-31.1, 26.05) -> (-31.1, 12.05)
  line L148 (-31.1, 12.05) -> (-45.1, 12.05)
  line L149 (-45.1, 12.05) -> (-45.1, 26.05)
  line L150 (-74.9438, 50.15) -> (-77.4625, 50.15)
  line L151 (-77.4625, 50.15) -> (-77.4625, 49.15)
  line L152 (-77.4625, 49.15) -> (-84.4625, 49.15)
  line L153 (-84.4625, 49.15) -> (-84.4625, 50.15)
  line L154 (-84.4625, 50.15) -> (-84.5745, 50.15)
  line L155 (-84.5745, 50.15) -> (-84.5745, 49.15)
  line L156 (-84.5745, 49.15) -> (-91.5745, 49.15)
  line L157 (-91.5745, 49.15) -> (-91.5745, 50.15)
  line L158 (-91.5745, 50.15) -> (-106.0375, 50.15)
  line L159 (-106.0375, 50.15) -> (-106.0375, 49.15)
  line L160 (-106.0375, 49.15) -> (-115.4505, 49.15)
  line L161 (-115.4505, 49.15) -> (-115.4505, 50.15)
  line L162 (-115.4505, 50.15) -> (-125.0558, 50.15)
  line L163 (-125.0557, 50.15) -> (-125.0557, 49.15)
  line L164 (-125.0557, 49.15) -> (-132.0875, 49.15)
  line L165 (-132.0875, 49.15) -> (-132.0875, 64.15)
  line L166 (-132.0875, 64.15) -> (-64.4375, 64.15)
  line L167 (-64.4375, 64.15) -> (-64.4375, 50.15)
  line L168 (-64.4375, 50.15) -> (-67.9375, 50.15)
  line L169 (-67.9375, 50.15) -> (-67.9375, 49.15)
  line L170 (-67.9375, 49.15) -> (-74.9438, 49.15)
  line L171 (-74.9438, 49.15) -> (-74.9438, 50.15)
  line L172 (-163.1875, 64.15) -> (-163.1875, 49.15)
  line L173 (-163.1875, 49.15) -> (-179.7125, 49.15)
  line L174 (-179.7125, 49.15) -> (-179.7125, 50.15)
  line L175 (-179.7125, 50.15) -> (-230.8375, 50.15)
  line L176 (-230.8375, 50.15) -> (-230.8375, 64.15)
  line L177 (-230.8375, 64.15) -> (-163.1875, 64.15)
  line L178 (-31.1, 45.1) -> (-31.1, 31.1)
  line L179 (-31.1, 31.1) -> (-45.1, 31.1)
  line L180 (-45.1, 31.1) -> (-45.1, 45.1)
  line L181 (-45.1, 45.1) -> (-31.1, 45.1)
  line L182 (-9.3813, 50.15) -> (-9.3813, 64.15)
  line L183 (-9.3813, 64.15) -> (4.6187, 64.15)
  line L184 (4.6187, 64.15) -> (4.6187, 50.15)
  line L185 (4.6187, 50.15) -> (-9.3813, 50.15)
  line L186 (-69.2, 31.1) -> (-83.2, 31.1)
  line L187 (-83.2, 31.1) -> (-83.2, 45.1)
  line L188 (-83.2, 45.1) -> (-69.2, 45.1)
  line L189 (-69.2, 45.1) -> (-69.2, 31.1)
  line L190 (-114.4438, -7) -> (-128.4437, -7)
  line L191 (-128.4437, -7) -> (-128.4437, 7)
  line L192 (-128.4437, 7) -> (-114.4438, 7)
  line L193 (-114.4438, 7) -> (-114.4438, -7)
  line L194 (7, 31.1) -> (-7, 31.1)
  line L195 (-7, 31.1) -> (-7, 45.1)
  line L196 (-7, 45.1) -> (7, 45.1)
  line L197 (7, 45.1) -> (7, 31.1)
  line L198 (-7, 26.05) -> (7, 26.05)
  line L199 (7, 26.05) -> (7, 12.05)
  line L200 (7, 12.05) -> (-7, 12.05)
  line L201 (-7, 12.05) -> (-7, 26.05)
  line L202 (-88.25, 45.1) -> (-88.25, 31.1)
  line L203 (-88.25, 31.1) -> (-102.25, 31.1)
  line L204 (-102.25, 31.1) -> (-102.25, 45.1)
  line L205 (-102.25, 45.1) -> (-88.25, 45.1)
  line L206 (-26.05, 31.1) -> (-26.05, 45.1)
  line L207 (-26.05, 45.1) -> (-12.05, 45.1)
  line L208 (-12.05, 45.1) -> (-12.05, 31.1)
  line L209 (-12.05, 31.1) -> (-26.05, 31.1)
  line L210 (-211.7875, 26.05) -> (-197.7875, 26.05)
  line L211 (-197.7875, 26.05) -> (-197.7875, 12.05)
  line L212 (-197.7875, 12.05) -> (-211.7875, 12.05)
  line L213 (-211.7875, 12.05) -> (-211.7875, 26.05)
sketch "plate_campsite" plane through (0, 10, 0) normal (0, 1, 0) x (-1, 0, 0)
  line L0 (-220.1576, -14) -> (-217.8482, -10)
  arc A0 (-216.1161, -9) -> (-217.8482, -10) centre (-216.1161, -11) ccw
  line L1 (-216.1161, -9) -> (-7.7214, -9)
  arc A1 (-5.9893, -10) -> (-7.7214, -9) centre (-7.7214, -11) ccw
  line L2 (-5.9893, -10) -> (-3.6799, -14)
  line L3 (-3.6799, -14) -> (4.3919, -14)
  line L4 (4.3919, -14) -> (6.7013, -10)
  arc A2 (8.4334, -9) -> (6.7013, -10) centre (8.4334, -11) ccw
  line L5 (8.4334, -9) -> (8.5, -9)
  arc A3 (8.5, -9) -> (9, -8.5) centre (8.5, -8.5) ccw
  line L6 (9, -8.5) -> (9, 65.65)
  arc A4 (9, 65.65) -> (8.5, 66.15) centre (8.5, 65.65) ccw
  line L7 (8.5, 66.15) -> (8.4334, 66.15)
  arc A5 (6.7013, 67.15) -> (8.4334, 66.15) centre (8.4334, 68.15) ccw
  line L8 (6.7013, 67.15) -> (4.3919, 71.15)
  line L9 (4.3919, 71.15) -> (-3.6799, 71.15)
  line L10 (-3.6799, 71.15) -> (-5.9893, 67.15)
  arc A6 (-7.7214, 66.15) -> (-5.9893, 67.15) centre (-7.7214, 68.15) ccw
  line L11 (-7.7214, 66.15) -> (-216.1161, 66.15)
  arc A7 (-217.8482, 67.15) -> (-216.1161, 66.15) centre (-216.1161, 68.15) ccw
  line L12 (-217.8482, 67.15) -> (-220.1576, 71.15)
  line L13 (-220.1576, 71.15) -> (-228.2294, 71.15)
  line L14 (-228.2294, 71.15) -> (-230.5388, 67.15)
  arc A8 (-232.2709, 66.15) -> (-230.5388, 67.15) centre (-232.2709, 68.15) ccw
  line L15 (-232.2709, 66.15) -> (-232.3375, 66.15)
  arc A9 (-232.3375, 66.15) -> (-232.8375, 65.65) centre (-232.3375, 65.65) ccw
  line L16 (-232.8375, 65.65) -> (-232.8375, -8.5)
  arc A10 (-232.8375, -8.5) -> (-232.3375, -9) centre (-232.3375, -8.5) ccw
  line L17 (-232.3375, -9) -> (-232.2709, -9)
  arc A11 (-230.5388, -10) -> (-232.2709, -9) centre (-232.2709, -11) ccw
  line L18 (-230.5388, -10) -> (-228.2294, -14)
  line L19 (-228.2294, -14) -> (-220.1576, -14)
  line L20 (-88.25, 26.05) -> (-88.25, 12.05)
  line L21 (-88.25, 12.05) -> (-102.25, 12.05)
  line L22 (-102.25, 12.05) -> (-102.25, 26.05)
  line L23 (-102.25, 26.05) -> (-88.25, 26.05)
  line L24 (-230.8375, 45.1) -> (-216.8375, 45.1)
  line L25 (-216.8375, 45.1) -> (-216.8375, 31.1)
  line L26 (-216.8375, 31.1) -> (-230.8375, 31.1)
  line L27 (-230.8375, 31.1) -> (-230.8375, 45.1)
  line L28 (-50.15, 31.1) -> (-64.15, 31.1)
  line L29 (-64.15, 31.1) -> (-64.15, 45.1)
  line L30 (-64.15, 45.1) -> (-50.15, 45.1)
  line L31 (-50.15, 45.1) -> (-50.15, 31.1)
  line L32 (-57.0063, 64.15) -> (-43.0063, 64.15)
  line L33 (-43.0063, 64.15) -> (-43.0063, 50.15)
  line L34 (-43.0063, 50.15) -> (-57.0063, 50.15)
  line L35 (-57.0063, 50.15) -> (-57.0063, 64.15)
  line L36 (-140.6375, 26.05) -> (-140.6375, 12.05)
  line L37 (-140.6375, 12.05) -> (-154.6375, 12.05)
  line L38 (-154.6375, 12.05) -> (-154.6375, 26.05)
  line L39 (-154.6375, 26.05) -> (-140.6375, 26.05)
  line L40 (-230.8375, -7) -> (-230.8375, 7)
  line L41 (-230.8375, 7) -> (-216.8375, 7)
  line L42 (-216.8375, 7) -> (-216.8375, -7)
  line L43 (-216.8375, -7) -> (-230.8375, -7)
  line L44 (-31.1, 7) -> (-31.1, -7)
  line L45 (-31.1, -7) -> (-45.1, -7)
  line L46 (-45.1, -7) -> (-45.1, 7)
  line L47 (-45.1, 7) -> (-31.1, 7)
  line L48 (-211.7875, 45.1) -> (-197.7875, 45.1)
  line L49 (-197.7875, 45.1) -> (-197.7875, 31.1)
  line L50 (-197.7875, 31.1) -> (-211.7875, 31.1)
  line L51 (-211.7875, 31.1) -> (-211.7875, 45.1)
  line L52 (-12.05, 26.05) -> (-12.05, 12.05)
  line L53 (-12.05, 12.05) -> (-26.05, 12.05)
  line L54 (-26.05, 12.05) -> (-26.05, 26.05)
  line L55 (-26.05, 26.05) -> (-12.05, 26.05)
  line L56 (-26.05, -7) -> (-26.05, 7)
  line L57 (-26.05, 7) -> (-12.05, 7)
  line L58 (-12.05, 7) -> (-12.05, -7)
  line L59 (-12.05, -7) -> (-26.05, -7)
  line L60 (-128.4437, 31.1) -> (-128.4437, 45.1)
  line L61 (-128.4437, 45.1) -> (-114.4438, 45.1)
  line L62 (-114.4438, 45.1) -> (-114.4438, 31.1)
  line L63 (-114.4438, 31.1) -> (-128.4437, 31.1)
  line L64 (-140.6375, 7) -> (-140.6375, -7)
  line L65 (-140.6375, -7) -> (-154.6375, -7)
  line L66 (-154.6375, -7) -> (-154.6375, 7)
  line L67 (-154.6375, 7) -> (-140.6375, 7)
  line L68 (-192.7375, 12.05) -> (-192.7375, 26.05)
  line L69 (-192.7375, 26.05) -> (-178.7375, 26.05)
  line L70 (-178.7375, 26.05) -> (-178.7375, 12.05)
  line L71 (-178.7375, 12.05) -> (-192.7375, 12.05)
  line L72 (-173.6875, 45.1) -> (-159.6875, 45.1)
  line L73 (-159.6875, 45.1) -> (-159.6875, 31.1)
  line L74 (-159.6875, 31.1) -> (-173.6875, 31.1)
  line L75 (-173.6875, 31.1) -> (-173.6875, 45.1)
  line L76 (-159.6875, -7) -> (-173.6875, -7)
  line L77 (-173.6875, -7) -> (-173.6875, 7)
  line L78 (-173.6875, 7) -> (-159.6875, 7)
  line L79 (-159.6875, 7) -> (-159.6875, -7)
  line L80 (-50.15, 26.05) -> (-50.15, 12.05)
  line L81 (-50.15, 12.05) -> (-64.15, 12.05)
  line L82 (-64.15, 12.05) -> (-64.15, 26.05)
  line L83 (-64.15, 26.05) -> (-50.15, 26.05)
  line L84 (-19.1938, 50.15) -> (-33.1938, 50.15)
  line L85 (-33.1938, 50.15) -> (-33.1938, 64.15)
  line L86 (-33.1938, 64.15) -> (-19.1938, 64.15)
  line L87 (-19.1938, 64.15) -> (-19.1938, 50.15)
  line L88 (-192.7375, 7) -> (-178.7375, 7)
  line L89 (-178.7375, 7) -> (-178.7375, -7)
  line L90 (-178.7375, -7) -> (-192.7375, -7)
  line L91 (-192.7375, -7) -> (-192.7375, 7)
  line L92 (-69.2, 7) -> (-69.2, -7)
  line L93 (-69.2, -7) -> (-83.2, -7)
  line L94 (-83.2, -7) -> (-83.2, 7)
  line L95 (-83.2, 7) -> (-69.2, 7)
  line L96 (-133.4938, 64.15) -> (-133.4938, 50.15)
  line L97 (-133.4938, 50.15) -> (-148.9318, 50.15)
  line L98 (-148.9317, 50.15) -> (-148.9317, 49.15)
  line L99 (-148.9317, 49.15) -> (-155.9317, 49.15)
  line L100 (-155.9317, 49.15) -> (-155.9317, 64.15)
  line L101 (-155.9317, 64.15) -> (-133.4938, 64.15)
  line L102 (-88.25, -7) -> (-102.25, -7)
  line L103 (-102.25, -7) -> (-102.25, 7)
  line L104 (-102.25, 7) -> (-88.25, 7)
  line L105 (-88.25, 7) -> (-88.25, -7)
  line L106 (-211.7875, 7) -> (-197.7875, 7)
  line L107 (-197.7875, 7) -> (-197.7875, -7)
  line L108 (-197.7875, -7) -> (-211.7875, -7)
  line L109 (-211.7875, -7) -> (-211.7875, 7)
  line L110 (-173.6875, 26.05) -> (-159.6875, 26.05)
  line L111 (-159.6875, 26.05) -> (-159.6875, 12.05)
  line L112 (-159.6875, 12.05) -> (-173.6875, 12.05)
  line L113 (-173.6875, 12.05) -> (-173.6875, 26.05)
  line L114 (-50.15, -7) -> (-64.15, -7)
  line L115 (-64.15, -7) -> (-64.15, 7)
  line L116 (-64.15, 7) -> (-50.15, 7)
  line L117 (-50.15, 7) -> (-50.15, -7)
  line L118 (-216.8375, 26.05) -> (-216.8375, 12.05)
  line L119 (-216.8375, 12.05) -> (-230.8375, 12.05)
  line L120 (-230.8375, 12.05) -> (-230.8375, 26.05)
  line L121 (-230.8375, 26.05) -> (-216.8375, 26.05)
  line L122 (-128.4437, 26.05) -> (-114.4438, 26.05)
  line L123 (-114.4438, 26.05) -> (-114.4438, 12.05)
  line L124 (-114.4438, 12.05) -> (-128.4437, 12.05)
  line L125 (-128.4437, 12.05) -> (-128.4437, 26.05)
  line L126 (-154.6375, 45.1) -> (-140.6375, 45.1)
  line L127 (-140.6375, 45.1) -> (-140.6375, 31.1)
  line L128 (-140.6375, 31.1) -> (-154.6375, 31.1)
  line L129 (-154.6375, 31.1) -> (-154.6375, 45.1)
  line L130 (-69.2, 12.05) -> (-83.2, 12.05)
  line L131 (-83.2, 12.05) -> (-83.2, 26.05)
  line L132 (-83.2, 26.05) -> (-69.2, 26.05)
  line L133 (-69.2, 26.05) -> (-69.2, 12.05)
  line L134 (-178.7375, 31.1) -> (-192.7375, 31.1)
  line L135 (-192.7375, 31.1) -> (-192.7375, 45.1)
  line L136 (-192.7375, 45.1) -> (-178.7375, 45.1)
  line L137 (-178.7375, 45.1) -> (-178.7375, 31.1)
  line L138 (7, -7) -> (-7, -7)
  line L139 (-7, -7) -> (-7, 7)
  line L140 (-7, 7) -> (7, 7)
  line L141 (7, 7) -> (7, -7)
  line L142 (-45.1, 26.05) -> (-31.1, 26.05)
  line L143 (-31.1, 26.05) -> (-31.1, 12.05)
  line L144 (-31.1, 12.05) -> (-45.1, 12.05)
  line L145 (-45.1, 12.05) -> (-45.1, 26.05)
  line L146 (-74.9438, 50.15) -> (-77.4625, 50.15)
  line L147 (-77.4625, 50.15) -> (-77.4625, 49.15)
  line L148 (-77.4625, 49.15) -> (-84.4625, 49.15)
  line L149 (-84.4625, 49.15) -> (-84.4625, 50.15)
  line L150 (-84.4625, 50.15) -> (-84.5745, 50.15)
  line L151 (-84.5745, 50.15) -> (-84.5745, 49.15)
  line L152 (-84.5745, 49.15) -> (-91.5745, 49.15)
  line L153 (-91.5745, 49.15) -> (-91.5745, 50.15)
  line L154 (-91.5745, 50.15) -> (-106.0375, 50.15)
  line L155 (-106.0375, 50.15) -> (-106.0375, 49.15)
  line L156 (-106.0375, 49.15) -> (-115.4505, 49.15)
  line L157 (-115.4505, 49.15) -> (-115.4505, 50.15)
  line L158 (-115.4505, 50.15) -> (-125.0558, 50.15)
  line L159 (-125.0557, 50.15) -> (-125.0557, 49.15)
  line L160 (-125.0557, 49.15) -> (-132.0875, 49.15)
  line L161 (-132.0875, 49.15) -> (-132.0875, 64.15)
  line L162 (-132.0875, 64.15) -> (-64.4375, 64.15)
  line L163 (-64.4375, 64.15) -> (-64.4375, 50.15)
  line L164 (-64.4375, 50.15) -> (-67.9375, 50.15)
  line L165 (-67.9375, 50.15) -> (-67.9375, 49.15)
  line L166 (-67.9375, 49.15) -> (-74.9438, 49.15)
  line L167 (-74.9438, 49.15) -> (-74.9438, 50.15)
  line L168 (-163.1875, 64.15) -> (-163.1875, 49.15)
  line L169 (-163.1875, 49.15) -> (-179.7125, 49.15)
  line L170 (-179.7125, 49.15) -> (-179.7125, 50.15)
  line L171 (-179.7125, 50.15) -> (-230.8375, 50.15)
  line L172 (-230.8375, 50.15) -> (-230.8375, 64.15)
  line L173 (-230.8375, 64.15) -> (-163.1875, 64.15)
  line L174 (-31.1, 45.1) -> (-31.1, 31.1)
  line L175 (-31.1, 31.1) -> (-45.1, 31.1)
  line L176 (-45.1, 31.1) -> (-45.1, 45.1)
  line L177 (-45.1, 45.1) -> (-31.1, 45.1)
  line L178 (-9.3813, 50.15) -> (-9.3813, 64.15)
  line L179 (-9.3813, 64.15) -> (4.6187, 64.15)
  line L180 (4.6187, 64.15) -> (4.6187, 50.15)
  line L181 (4.6187, 50.15) -> (-9.3813, 50.15)
  line L182 (-69.2, 31.1) -> (-83.2, 31.1)
  line L183 (-83.2, 31.1) -> (-83.2, 45.1)
  line L184 (-83.2, 45.1) -> (-69.2, 45.1)
  line L185 (-69.2, 45.1) -> (-69.2, 31.1)
  line L186 (-114.4438, -7) -> (-128.4437, -7)
  line L187 (-128.4437, -7) -> (-128.4437, 7)
  line L188 (-128.4437, 7) -> (-114.4438, 7)
  line L189 (-114.4438, 7) -> (-114.4438, -7)
  line L190 (7, 31.1) -> (-7, 31.1)
  line L191 (-7, 31.1) -> (-7, 45.1)
  line L192 (-7, 45.1) -> (7, 45.1)
  line L193 (7, 45.1) -> (7, 31.1)
  line L194 (-7, 26.05) -> (7, 26.05)
  line L195 (7, 26.05) -> (7, 12.05)
  line L196 (7, 12.05) -> (-7, 12.05)
  line L197 (-7, 12.05) -> (-7, 26.05)
  line L198 (-88.25, 45.1) -> (-88.25, 31.1)
  line L199 (-88.25, 31.1) -> (-102.25, 31.1)
  line L200 (-102.25, 31.1) -> (-102.25, 45.1)
  line L201 (-102.25, 45.1) -> (-88.25, 45.1)
  line L202 (-26.05, 31.1) -> (-26.05, 45.1)
  line L203 (-26.05, 45.1) -> (-12.05, 45.1)
  line L204 (-12.05, 45.1) -> (-12.05, 31.1)
  line L205 (-12.05, 31.1) -> (-26.05, 31.1)
  line L206 (-211.7875, 26.05) -> (-197.7875, 26.05)
  line L207 (-197.7875, 26.05) -> (-197.7875, 12.05)
  line L208 (-197.7875, 12.05) -> (-211.7875, 12.05)
  line L209 (-211.7875, 12.05) -> (-211.7875, 26.05)